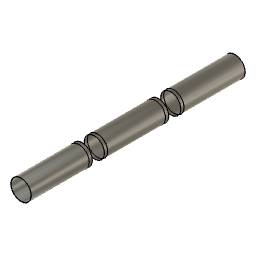
final tube rocket v3 (Autodesk Fusion 360 design; units mm, degrees)
Autodesk Fusion 360 part; units mm, degrees
sketch "Sketch1" plane through (0, 0, 0) normal (0, 1, 0) x (1, 0, 0)
  circle A0 centre (0, 0) radius 33.5
  circle A1 centre (0, 0) radius 29.5
  dimension "d1" = 67
  dimension "d2" = 59
  constraint coincident A0.centre A1.centre
  constraint concentric A0 A1
  measures "d1" diameter of A0
  measures "d2" diameter of A1
extrude "Extrude1" add sketch "Sketch1" along normal blind 800 makes body 1
ref_plane "WorkPlane1" through (0, 200, 0) normal (0, 1, 0) x (0, 0, 1)
ref_plane "WorkPlane2" through (0, 400, 0) normal (0, 1, 0) x (0, 0, 1)
ref_plane "WorkPlane3" through (0, 600, 0) normal (0, 1, 0) x (0, 0, 1)
extrude "Extrude2" cut 1 faces at (31.9321, 800, 3.1299) along direction (0, -1, 0) blind 200 on bodies 1 bodies 1
split "Split1" by plane through (0, 200, 0) normal (0, 1, 0) bodies 1 makes body 2 at (33.3335, 333.3333, -3.3355)
split "Split2" by plane through (0, 400, 0) normal (0, 1, 0) bodies 2 makes body 3 at (33.3335, 466.6667, -3.3355)
move_body "Move1" bodies 3 to x (1, 0, 0) y (0, 1, 0) z (0, 0, 1) at (0, 200, 0)
move_body "Move2" bodies 2 to x (1, 0, 0) y (0, 1, 0) z (0, 0, 1) at (0, 100, 0)
sketch "Sketch2" plane through (0, 200, 0) normal (0, 1, 0) x (-1, 0, 0)
  circle A0 centre (0, 0) radius 29.5
  circle A1 centre (0, 0) radius 33.5
  circle A2 centre (0, 0) radius 31.5
  dimension "d10" = 63
  constraint coincident A0.centre A1.centre
  measures "d10" diameter of A2
extrude "Extrude3" cut sketch "Sketch2" against normal blind 10 contours A2 bodies 1
sketch "Sketch3" plane through (0, 300, 0) normal (0, -1, 0) x (1, 0, 0)
  circle A0 centre (0, 0) radius 33.5
  circle A1 centre (0, 0) radius 29.5
  circle A2 centre (0, 0) radius 31.5
  dimension "d13" = 63
  constraint concentric A0 A2
  measures "d13" diameter of A2
extrude "Extrude4" add sketch "Sketch3" along normal blind 10 contours A2 bodies 2
sketch "Sketch4" plane through (0, 500, 0) normal (0, 1, 0) x (-1, 0, 0)
  circle A0 centre (0, 0) radius 29.5
  circle A1 centre (0, 0) radius 33.5
  circle A2 centre (0, 0) radius 31.5
  dimension "d16" = 63
  constraint coincident A0.centre A1.centre
  measures "d16" diameter of A2
extrude "Extrude5" cut sketch "Sketch4" against normal blind 10 contours A2 bodies 2
sketch "Sketch5" plane through (0, 600, 0) normal (0, -1, 0) x (1, 0, 0)
  circle A0 centre (0, 0) radius 33.5
  circle A1 centre (0, 0) radius 29.5
  circle A2 centre (0, 0) radius 31.5
  dimension "d19" = 63
  constraint coincident A0.centre A1.centre
  measures "d19" diameter of A2
extrude "Extrude6" add sketch "Sketch5" along normal blind 10 contours A2 bodies 3
move_body "Move3" bodies 2 to x (1, 0, 0) y (0, 1, 0) z (0, 0, 1) at (0, -100, 0)
move_body "Move4" bodies 3 to x (1, 0, 0) y (0, 1, 0) z (0, 0, 1) at (0, -200, 0)
sketch "Sketch7" plane through (0, 0, 0) normal (0, 1, 0) x (1, 0, 0)
  circle A0 centre (0, 0) radius 32.5
  dimension "d22" = 65
  constraint coincident A0.centre origin
  measures "d22" diameter of A0
extrude "Extrude7" cut sketch "Sketch7" along normal blind 610 bodies 1 2 3
move_body "Move5" bodies 3 to x (1, 0, 0) y (0, 1, 0) z (0, 0, 1) at (0, 100, 0)
move_body "Move6" bodies 3 to x (1, 0, 0) y (0, 1, 0) z (0, 0, 1) at (0, 100, 0)
move_body "Move7" bodies 2 to x (1, 0, 0) y (0, 1, 0) z (0, 0, 1) at (0, 100, 0)
sketch "Sketch8" plane through (0, 200, 0) normal (0, 1, 0) x (-1, 0, 0)
  circle A0 centre (0, 0) radius 32.5
  circle A1 centre (0, 0) radius 33.5
  circle A2 centre (0, 0) radius 33
  dimension "d25" = 66
  constraint coincident A0.centre A1.centre
  measures "d25" diameter of A2
extrude "Extrude8" cut sketch "Sketch8" against normal blind 10 contours A2 bodies 1
sketch "Sketch9" plane through (0, 300, 0) normal (0, -1, 0) x (1, 0, 0)
  circle A0 centre (0, 0) radius 32.5
  circle A1 centre (0, 0) radius 33.5
  circle A2 centre (0, 0) radius 33
  dimension "d28" = 66
  constraint coincident A0.centre A1.centre
  measures "d28" diameter of A2
extrude "Extrude9" add sketch "Sketch9" along normal blind 10 contours A2 bodies 2
sketch "Sketch10" plane through (0, 500, 0) normal (0, 1, 0) x (-1, 0, 0)
  circle A0 centre (0, 0) radius 32.5
  circle A1 centre (0, 0) radius 33.5
  circle A2 centre (0, 0) radius 33
  dimension "d31" = 66
  constraint coincident A0.centre A1.centre
  measures "d31" diameter of A2
extrude "Extrude10" cut sketch "Sketch10" against normal blind 10 contours A2 bodies 2
sketch "Sketch11" plane through (0, 600, 0) normal (0, -1, 0) x (1, 0, 0)
  circle A0 centre (0, 0) radius 32.5
  circle A1 centre (0, 0) radius 33.5
  circle A2 centre (0, 0) radius 33
  dimension "d34" = 66
  constraint coincident A0.centre A1.centre
  measures "d34" diameter of A2
extrude "Extrude11" add sketch "Sketch11" along normal blind 10 contours A2 bodies 3
move_body "Move8" bodies 2 to x (1, 0, 0) y (0, 1, 0) z (0, 0, 1) at (0, 100, 0)
move_body "Move9" bodies 1 to x (1, 0, 0) y (0, 1, 0) z (0, 0, 1) at (0, 200, 0)
move_body "Move10" bodies 1 to x (1, 0, 0) y (0, 1, 0) z (0, 0, 1) at (0, -50, 0)
move_body "Move11" bodies 1 to x (1, 0, 0) y (0, 1, 0) z (0, 0, 1) at (0, -50, 0)
move_body "Move12" bodies 2 to x (1, 0, 0) y (0, 1, 0) z (0, 0, 1) at (0, -50, 0)
sketch "Sketch12" plane through (0, 0, 0) normal (0, 1, 0) x (1, 0, 0)
  circle A0 centre (0, 0) radius 32.5
  circle A1 centre (0, 0) radius 33.5
  dimension "d37" = 65
  dimension "d38" = 67
  measures "d37" diameter of A0
  measures "d38" diameter of A1
sketch "Sketch6" plane through (0, 0, 0) normal (0, 0, 1) x (1, 0, 0)
equation "d2 = 67 mm - 8 mm"
